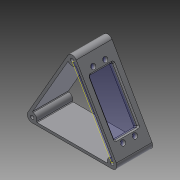
# Autodesk Inventor part: ServoHousing
Saved by Autodesk Inventor 2014 SP1 (Build 180222100, 222)
## iProperties
Created: 2014-11-03
Part Number: ServoHousing
Material: Generic
Document SubType Name: Modeling
Designer: rawrdong
Density: 1 g/cm^3
Appearance: Default
Author: rawrdong
Autodesk Inventor part; units mm, degrees
ref_plane "YZ Plane" through (0, 0, 0) normal (1, 0, 0) x (0, 1, 0)
ref_plane "XZ Plane" through (0, 0, 0) normal (0, 1, 0) x (-1, 0, 0)
ref_plane "XY Plane" through (0, 0, 0) normal (0, 0, 1) x (1, 0, 0)
sketch "Sketch2" plane through (0, 0, 0) normal (0, 1, 0) x (-1, 0, 0)
  circle A0 centre (0, 38.6825) radius 1.425
  circle A1 centre (0, 38.6825) radius 4
  circle A2 centre (-33.5, -19.3412) radius 1.425
  circle A3 centre (-33.5, -19.3412) radius 4
  circle A4 centre (33.5, -19.3412) radius 1.425
  circle A5 centre (33.5, -19.3412) radius 4
  line L0 (-36.9641, -17.3412) -> (-3.4641, 40.6825)
  line L1 (-3.314, 36.4425) -> (-33.2171, -15.3513)
  line L2 (-33.5, -23.3412) -> (33.5, -23.3412)
  line L3 (36.9641, -17.3412) -> (3.4641, 40.6825)
  line L4 (-29.9031, -21.0912) -> (29.9031, -21.0912)
  line L5 (33.2171, -15.3513) -> (3.314, 36.4425)
  line L6 (0, -23.3412) -> (0, -21.0912) construction
  line L7 (20.2141, 11.6706) -> (18.2655, 10.5456) construction
  line L8 (-18.2655, 10.5456) -> (-20.2141, 11.6706) construction
  point P0 (0, 0)
  point P1 (0, 0)
  dimension "d21" = 360
  dimension "d23" = 67
  dimension "d24" = 2.85
  dimension "d25" = 8
  dimension "d30" = 2.25
  constraints: 18 end point, 12 point on circle, 6 centre point, 6 midpoint, 6 tangent, 4 coincident, 3 parallel, 2 equal length, 1 horizontal, 1 vertical alignment, 13 other
  measures "d23" distance of A4.centre A2.centre
  measures "d24" diameter of A2
  measures "d25" diameter of A3
  measures "d30" distance between parallel lines of L0 L1
extrude "Extrusion3" add sketch "Sketch2" along normal blind 30 contours A1 | A1 L3 A5 L5 | A1 L1 A3 L0 | A5 | A3 | A5 L2 A3 L4
sketch "Servo1" plane through (36.9641, 0, -17.3412) normal (0.8660254, 0, 0.5) x (0.5, 0, -0.8660254)
  line L0 (-67, 30) -> (0, 30) projected
  line L1 (-54.5, 24.75) -> (-12.5, 24.75)
  line L2 (-12.5, 24.75) -> (-12.5, 5.25)
  line L3 (-12.5, 5.25) -> (-54.5, 5.25)
  line L4 (-54.5, 5.25) -> (-54.5, 24.75)
  circle A0 centre (-8.6975, 20.025) radius 2.025
  circle A1 centre (-8.6975, 9.975) radius 2.025
  line L5 (-33.5, 30) -> (-33.5, -15.5284)
  line L6 (-12.5, 15) -> (-54.5, 15) construction
  circle A2 centre (-58.3025, 20.025) radius 2.025
  circle A3 centre (-58.3025, 9.975) radius 2.025
  line L7 (0, 0) -> (0, 30) projected
  point P0 (-33.5, 0)
  point P1 (-33.5, 5.25)
  point P2 (0, 15)
  dimension "d43" = 4.05
  dimension "d44" = 19.5
  dimension "d45" = 42
  dimension "d46" = 6
  dimension "d47" = 49.605
  constraints: 12 end point, 5 midpoint, 4 centre point, 3 parallel, 3 symmetric about line, 1 equal radius, 1 horizontal, 1 horizontal alignment, 1 perpendicular, 1 point on line, 2 other
  measures "d43" diameter of A0
  measures "d44" distance of L3.end L1.start
  measures "d45" distance of L2.end L3.end
  measures "d47" diameter of A0.centre L5
extrude "Extrusion4" cut sketch "Servo1" against normal blind 27 contours L1 L5 L3 L4 | L1 L2 L3 L5
extrude "Extrusion5" cut sketch "Servo1" against normal up to next contours A0 | A1 | A2 | A3
fillet "Fillet4" radius 0.8 4 edges at (8.7398, 24.75, 29.2947) (8.7398, 5.25, 29.2947) (29.7398, 5.25, -7.0784) (29.7398, 24.75, -7.0784)
ref_plane "Work Plane1" through (3.314, 0, 36.4425) normal (-0.8660254, 0, -0.5) x (-0.5, 0, 0.8660254)
sketch "Sketch7" plane through (3.314, 0, 36.4425) normal (-0.8660254, 0, -0.5) x (-0.5, 0, 0.8660254)
  line L0 (-8.9031, 6.05) -> (-8.9031, 23.95) projected
  line L1 (-9.7031, 24.75) -> (-50.1031, 24.75) projected
  arc A0 (-8.9031, 23.95) -> (-9.7031, 24.75) centre (-9.7031, 23.95) ccw projected
  arc A1 (-9.7031, 5.25) -> (-8.9031, 6.05) centre (-9.7031, 6.05) ccw projected
  line L2 (-50.1031, 5.25) -> (-9.7031, 5.25) projected
  arc A2 (-50.9031, 6.05) -> (-50.1031, 5.25) centre (-50.1031, 6.05) ccw projected
  line L3 (-50.9031, 23.95) -> (-50.9031, 6.05) projected
  arc A3 (-50.1031, 24.75) -> (-50.9031, 23.95) centre (-50.1031, 23.95) ccw projected
  line L4 (-50.1031, 27.25) -> (-9.7031, 27.25)
  arc A4 (-6.4031, 23.95) -> (-9.7031, 27.25) centre (-9.7031, 23.95) ccw
  line L5 (-6.4031, 23.95) -> (-6.4031, 6.05)
  arc A5 (-9.7031, 2.75) -> (-6.4031, 6.05) centre (-9.7031, 6.05) ccw
  line L6 (-9.7031, 2.75) -> (-50.1031, 2.75)
  arc A6 (-53.4031, 6.05) -> (-50.1031, 2.75) centre (-50.1031, 6.05) ccw
  line L7 (-53.4031, 6.05) -> (-53.4031, 23.95)
  arc A7 (-50.1031, 27.25) -> (-53.4031, 23.95) centre (-50.1031, 23.95) ccw
  line L8 (-53.4031, 23.95) -> (-62.349, 23.95)
  line L9 (-62.349, 23.95) -> (-62.349, 6.05)
  line L10 (-53.4031, 6.05) -> (-62.349, 6.05)
  line L11 (-29.9031, 5.25) -> (-29.9031, 24.75) construction
  line L12 (-6.4031, 23.95) -> (2.5428, 23.95)
  line L13 (2.5428, 23.95) -> (2.5428, 6.05)
  line L14 (-6.4031, 6.05) -> (2.5428, 6.05)
  circle A8 centre (-54.7056, 20.025) radius 2.025 projected
  circle A9 centre (-54.7056, 9.975) radius 2.025 projected
  circle A10 centre (-5.1006, 9.975) radius 2.025 projected
  circle A11 centre (-5.1006, 20.025) radius 2.025 projected
  dimension "d82" = 2.5
  constraints: 22 end point, 8 point on circle, 4 centre point, 3 perpendicular, 2 horizontal, 2 midpoint, 1 vertical, 8 other
  measures "d82" distance between parallel lines of L4 L1
extrude "Extrusion8" add sketch "Sketch7" along normal blind 2 contours L4 A4 L5 A11 A10 A5 L6 A6 L7 A9 A8 A7 | L7 A8 A9 L10 L9 L8 | L12 L13 L14 L5 A10 A11
fillet "Fillet6" radius 2 4 edges at (29.1495, 23.95, -10.306) (5.6495, 23.95, 30.3972) (5.6495, 6.05, 30.3972) (29.1495, 6.05, -10.306)
chamfer "Chamfer2" distance 2 angle 45 14 edges at (18.2655, 27.25, 10.5456) (7.2449, 26.6886, 29.6339) (6.2694, 24.2903, 31.3235) (4.5127, 23.95, 34.3662) (29.2862, 26.6886, -8.5427) (30.2617, 24.2903, -10.2323) (32.0184, 23.95, -13.275) (18.2655, 2.75, 10.5456) (29.2862, 3.3114, -8.5427) (30.2617, 5.7097, -10.2323) (32.0184, 6.05, -13.275) (7.2449, 3.3114, 29.6339) (6.2694, 5.7097, 31.3235) (4.5127, 6.05, 34.3662)
fillet "Fillet7" radius 0.5 8 edges at (3.314, 2.0251, 36.4425) (-3.314, 15, 36.4425) (3.314, 27.975, 36.4425) (-33.2171, 15, -15.3513) (-29.9031, 15, -21.0912) (29.9031, 15, -21.0912) (33.2171, 2.025, -15.3513) (33.2171, 27.9749, -15.3513)
chamfer "Chamfer3" distance 1 angle 45 8 edges at (20.2141, 5.25, 11.6706) (9.8313, 5.4843, 29.6542) (9.7141, 15, 29.8572) (9.8313, 24.5157, 29.6542) (20.2141, 24.75, 11.6706) (30.5969, 24.5157, -6.313) (30.7141, 15, -6.5159) (30.5969, 5.4843, -6.313)
body "Solid2"
body "Solid3"
